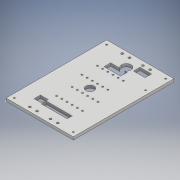
# Autodesk Inventor part: 一枚目2018.8.7
Saved by Autodesk Inventor 2018 (Build 220112000, 112)
## iProperties
Created: 2018-08-07
Part Number: 一枚目2018.8.7
Material: 一般
Document SubType Name: Modeling
Designer: shun2
Density: 1 g/cm^3
Appearance: 既定
Author: shun2
Autodesk Inventor part; units mm, degrees
(part 1 of 2)
ref_plane "YZ Plane" through (0, 0, 0) normal (1, 0, 0) x (0, 1, 0)
ref_plane "XZ Plane" through (0, 0, 0) normal (0, 1, 0) x (-1, 0, 0)
ref_plane "XY Plane" through (0, 0, 0) normal (0, 0, 1) x (1, 0, 0)
sketch "スケッチ1" plane through (0, 0, 0) normal (0, 0, 1) x (1, 0, 0)
  line L0 (0, 0) -> (130, 0)
  line L1 (130, 0) -> (130, 194.7239)
  line L2 (130, 194.7239) -> (0, 194.7239)
  line L3 (0, 194.7239) -> (0, 0)
  circle A0 centre (78, 186.7239) radius 2.15
  circle A1 centre (92, 186.7239) radius 2.15
  circle A2 centre (52, 186.7239) radius 2.15
  circle A3 centre (38, 186.7239) radius 2.15
  circle A4 centre (78, 8) radius 2.15
  circle A5 centre (92, 8) radius 2.15
  circle A6 centre (52, 8) radius 2.15
  circle A7 centre (38, 8) radius 2.15
  circle A8 centre (95.5, 52.362) radius 1.6
  circle A9 centre (45.5, 52.362) radius 1.6
  circle A10 centre (55.5, 52.362) radius 1.6
  circle A11 centre (65.5, 52.362) radius 1.6
  circle A12 centre (75.5, 52.362) radius 1.6
  circle A13 centre (85.5, 52.362) radius 1.6
  circle A14 centre (95.5, 82.362) radius 1.6
  circle A15 centre (45.5, 82.362) radius 1.6
  circle A16 centre (55.5, 82.362) radius 1.6
  circle A17 centre (65.5, 82.362) radius 1.6
  circle A18 centre (75.5, 82.362) radius 1.6
  circle A19 centre (85.5, 82.362) radius 1.6
  circle A20 centre (34.5, 142.362) radius 1.6
  circle A21 centre (84.5, 142.362) radius 1.6
  circle A22 centre (74.5, 142.362) radius 1.6
  circle A23 centre (64.5, 142.362) radius 1.6
  circle A24 centre (54.5, 142.362) radius 1.6
  circle A25 centre (44.5, 142.362) radius 1.6
  circle A26 centre (34.5, 112.362) radius 1.6
  circle A27 centre (84.5, 112.362) radius 1.6
  circle A28 centre (74.5, 112.362) radius 1.6
  circle A29 centre (64.5, 112.362) radius 1.6
  circle A30 centre (54.5, 112.362) radius 1.6
  circle A31 centre (44.5, 112.362) radius 1.6
  circle A32 centre (65, 97.362) radius 8
  arc A33 (69.6765, 160.0343) -> (60.3235, 160.0343) centre (65, 167.7239) ccw
  circle A34 centre (122, 8) radius 1.6
  circle A35 centre (8, 186.7239) radius 1.6
  circle A36 centre (122, 186.7239) radius 1.6
  circle A37 centre (8, 8) radius 1.6
  circle A38 centre (122, 147.7239) radius 1.6
  line L4 (65, 197.7239) -> (65, -3)
  line L5 (-3, 97.362) -> (133, 97.362)
  line L6 (8, 182.1239) -> (8, 191.3239)
  line L7 (117.4, 186.7239) -> (126.6, 186.7239)
  line L8 (122, 182.1239) -> (122, 191.3239)
  line L9 (117.4, 8) -> (126.6, 8)
  line L10 (3.4, 186.7239) -> (12.6, 186.7239)
  line L11 (122, 3.4) -> (122, 12.6)
  line L12 (3.4, 8) -> (12.6, 8)
  line L13 (8, 3.4) -> (8, 12.6)
  line L14 (117.4, 147.7239) -> (126.6, 147.7239)
  line L15 (122, 143.1239) -> (122, 152.3239)
  arc A39 (69.6765, 160.0343) -> (65, 176.7239) centre (65, 167.7239) ccw
  arc A40 (65, 176.7239) -> (60.3235, 160.0343) centre (65, 167.7239) ccw
  line L16 (83.4433, 173.4847) -> (95.4433, 173.4847)
  arc A41 (95.4433, 173.453) -> (95.4433, 173.5164) centre (95.4433, 173.4847) ccw
  arc A42 (83.4433, 173.5164) -> (83.4433, 173.453) centre (83.4433, 173.4847) ccw
  line L17 (95.4433, 173.4847) -> (95.4433, 176.9847)
  arc A43 (95.4751, 176.9847) -> (95.4116, 176.9847) centre (95.4434, 176.9847) ccw
  arc A44 (95.4116, 173.4847) -> (95.4751, 173.4847) centre (95.4434, 173.4847) ccw
  line L18 (95.4433, 176.9847) -> (83.4433, 176.9847)
  arc A45 (83.4433, 177.0164) -> (83.4433, 176.953) centre (83.4433, 176.9847) ccw
  arc A46 (95.4433, 176.953) -> (95.4433, 177.0164) centre (95.4433, 176.9847) ccw
  line L19 (83.4433, 176.9847) -> (83.4433, 173.4847)
  arc A47 (83.4116, 173.4847) -> (83.4751, 173.4847) centre (83.4434, 173.4847) ccw
  arc A48 (83.4751, 176.9847) -> (83.4116, 176.9847) centre (83.4434, 176.9847) ccw
  line L20 (56.515, 150.7744) -> (56.515, 152.1714)
  arc A49 (56.5531, 152.1714) -> (56.4769, 152.1714) centre (56.515, 152.1714) ccw
  arc A50 (56.4769, 150.7744) -> (56.5531, 150.7744) centre (56.515, 150.7744) ccw
  line L21 (46.355, 158.2674) -> (56.515, 158.2674)
  arc A51 (56.515, 158.2293) -> (56.515, 158.3055) centre (56.515, 158.2674) ccw
  arc A52 (46.355, 158.3055) -> (46.355, 158.2293) centre (46.355, 158.2674) ccw
  line L22 (46.355, 158.2674) -> (46.355, 156.4894)
  arc A53 (46.3169, 156.4894) -> (46.3931, 156.4894) centre (46.355, 156.4894) ccw
  arc A54 (46.3931, 158.2674) -> (46.3169, 158.2674) centre (46.355, 158.2674) ccw
  line L23 (56.515, 150.7744) -> (46.355, 150.7744)
  arc A55 (46.355, 150.8125) -> (46.355, 150.7363) centre (46.355, 150.7744) ccw
  arc A56 (56.515, 150.7363) -> (56.515, 150.8125) centre (56.515, 150.7744) ccw
  line L24 (56.515, 157.3784) -> (57.023, 157.5054)
  arc A57 (57.0322, 157.4684) -> (57.0138, 157.5424) centre (57.023, 157.5054) ccw
  arc A58 (56.5058, 157.4154) -> (56.5242, 157.3414) centre (56.515, 157.3784) ccw
  line L25 (56.515, 157.3784) -> (56.515, 158.2674)
  arc A59 (56.5531, 158.2674) -> (56.4769, 158.2674) centre (56.515, 158.2674) ccw
  arc A60 (56.4769, 157.3784) -> (56.5531, 157.3784) centre (56.515, 157.3784) ccw
  line L26 (57.023, 157.5054) -> (57.023, 156.3624)
  arc A61 (56.9849, 156.3624) -> (57.0611, 156.3624) centre (57.023, 156.3624) ccw
  arc A62 (57.0611, 157.5054) -> (56.9849, 157.5054) centre (57.023, 157.5054) ccw
  line L27 (57.023, 156.3624) -> (56.515, 156.4894)
  arc A63 (56.5242, 156.5264) -> (56.5058, 156.4524) centre (56.515, 156.4894) ccw
  arc A64 (57.0138, 156.3254) -> (57.0322, 156.3994) centre (57.023, 156.3624) ccw
  line L28 (56.515, 156.4894) -> (56.515, 157.3784)
  arc A65 (56.5531, 157.3784) -> (56.4769, 157.3784) centre (56.515, 157.3784) ccw
  arc A66 (56.4769, 156.4894) -> (56.5531, 156.4894) centre (56.515, 156.4894) ccw
  line L29 (56.515, 156.4894) -> (46.355, 156.4894)
  arc A67 (46.355, 156.5275) -> (46.355, 156.4513) centre (46.355, 156.4894) ccw
  arc A68 (56.515, 156.4513) -> (56.515, 156.5275) centre (56.515, 156.4894) ccw
  line L30 (46.355, 156.4894) -> (46.355, 152.1714)
  arc A69 (46.3169, 152.1714) -> (46.3931, 152.1714) centre (46.355, 152.1714) ccw
  arc A70 (46.3931, 156.4894) -> (46.3169, 156.4894) centre (46.355, 156.4894) ccw
  line L31 (56.515, 152.1714) -> (46.355, 152.1714)
  arc A71 (46.355, 152.2095) -> (46.355, 152.1333) centre (46.355, 152.1714) ccw
  arc A72 (56.515, 152.1333) -> (56.515, 152.2095) centre (56.515, 152.1714) ccw
  line L32 (56.515, 152.1714) -> (56.515, 156.4894)
  arc A73 (56.5531, 156.4894) -> (56.4769, 156.4894) centre (56.515, 156.4894) ccw
  arc A74 (56.4769, 152.1714) -> (56.5531, 152.1714) centre (56.515, 152.1714) ccw
  line L33 (46.355, 152.1714) -> (46.355, 150.7744)
  arc A75 (46.3169, 150.7744) -> (46.3931, 150.7744) centre (46.355, 150.7744) ccw
  arc A76 (46.3931, 152.1714) -> (46.3169, 152.1714) centre (46.355, 152.1714) ccw
  line L34 (60.565, 151.81) -> (60.565, 156.89)
  arc A77 (60.5968, 156.89) -> (60.5333, 156.89) centre (60.5651, 156.89) ccw
  arc A78 (60.5333, 151.81) -> (60.5968, 151.81) centre (60.5651, 151.81) ccw
  line L35 (60.565, 156.89) -> (61.835, 156.89)
  arc A79 (61.835, 156.8583) -> (61.835, 156.9218) centre (61.835, 156.8901) ccw
  arc A80 (60.565, 156.9218) -> (60.565, 156.8583) centre (60.565, 156.8901) ccw
  line L36 (61.835, 156.89) -> (69.455, 156.89)
  arc A81 (69.455, 156.8583) -> (69.455, 156.9218) centre (69.455, 156.8901) ccw
  arc A82 (61.835, 156.9218) -> (61.835, 156.8583) centre (61.835, 156.8901) ccw
  line L37 (69.455, 156.89) -> (70.725, 156.89)
  arc A83 (70.725, 156.8583) -> (70.725, 156.9218) centre (70.725, 156.8901) ccw
  arc A84 (69.455, 156.9218) -> (69.455, 156.8583) centre (69.455, 156.8901) ccw
  line L38 (70.725, 156.89) -> (70.725, 151.81)
  arc A85 (70.6933, 151.81) -> (70.7568, 151.81) centre (70.725, 151.81) ccw
  arc A86 (70.7568, 156.89) -> (70.6933, 156.89) centre (70.725, 156.89) ccw
  line L39 (70.725, 151.81) -> (60.565, 151.81)
  arc A87 (60.565, 151.8417) -> (60.565, 151.7783) centre (60.565, 151.81) ccw
  arc A88 (70.725, 151.7783) -> (70.725, 151.8417) centre (70.725, 151.81) ccw
  line L40 (61.835, 156.89) -> (61.835, 155.62)
  arc A89 (61.8032, 155.62) -> (61.8668, 155.62) centre (61.835, 155.62) ccw
  arc A90 (61.8668, 156.89) -> (61.8032, 156.89) centre (61.835, 156.89) ccw
  line L41 (61.835, 155.62) -> (69.455, 155.62)
  arc A91 (69.455, 155.5883) -> (69.455, 155.6517) centre (69.455, 155.62) ccw
  arc A92 (61.835, 155.6517) -> (61.835, 155.5883) centre (61.835, 155.62) ccw
  line L42 (69.455, 155.62) -> (69.455, 156.89)
  arc A93 (69.4868, 156.89) -> (69.4232, 156.89) centre (69.455, 156.89) ccw
  arc A94 (69.4232, 155.62) -> (69.4868, 155.62) centre (69.455, 155.62) ccw
  arc A95 (93.9433, 174.5922) -> (93.9433, 175.1172) centre (93.9433, 174.8547) ccw
  arc A96 (93.9433, 175.1172) -> (93.9433, 174.5922) centre (93.9433, 174.8547) ccw
  arc A97 (93.9433, 174.5922) -> (93.9433, 175.1172) centre (93.9433, 174.8547) ccw
  arc A98 (93.9433, 175.1172) -> (93.9433, 174.5922) centre (93.9433, 174.8547) ccw
  arc A99 (92.4433, 174.5922) -> (92.4433, 175.1172) centre (92.4433, 174.8547) ccw
  arc A100 (92.4433, 175.1172) -> (92.4433, 174.5922) centre (92.4433, 174.8547) ccw
  arc A101 (92.4433, 174.5922) -> (92.4433, 175.1172) centre (92.4433, 174.8547) ccw
  arc A102 (92.4433, 175.1172) -> (92.4433, 174.5922) centre (92.4433, 174.8547) ccw
  arc A103 (90.9433, 174.5922) -> (90.9433, 175.1172) centre (90.9433, 174.8547) ccw
  arc A104 (90.9433, 175.1172) -> (90.9433, 174.5922) centre (90.9433, 174.8547) ccw
  arc A105 (90.9433, 174.5922) -> (90.9433, 175.1172) centre (90.9433, 174.8547) ccw
  arc A106 (90.9433, 175.1172) -> (90.9433, 174.5922) centre (90.9433, 174.8547) ccw
  arc A107 (89.4433, 174.5922) -> (89.4433, 175.1172) centre (89.4433, 174.8547) ccw
  arc A108 (89.4433, 175.1172) -> (89.4433, 174.5922) centre (89.4433, 174.8547) ccw
  arc A109 (89.4433, 174.5922) -> (89.4433, 175.1172) centre (89.4433, 174.8547) ccw
  arc A110 (89.4433, 175.1172) -> (89.4433, 174.5922) centre (89.4433, 174.8547) ccw
  arc A111 (87.9433, 174.5922) -> (87.9433, 175.1172) centre (87.9433, 174.8547) ccw
  arc A112 (87.9433, 175.1172) -> (87.9433, 174.5922) centre (87.9433, 174.8547) ccw
  arc A113 (87.9433, 174.5922) -> (87.9433, 175.1172) centre (87.9433, 174.8547) ccw
  arc A114 (87.9433, 175.1172) -> (87.9433, 174.5922) centre (87.9433, 174.8547) ccw
  arc A115 (86.4433, 174.5922) -> (86.4433, 175.1172) centre (86.4433, 174.8547) ccw
  arc A116 (86.4433, 175.1172) -> (86.4433, 174.5922) centre (86.4433, 174.8547) ccw
  arc A117 (86.4433, 174.5922) -> (86.4433, 175.1172) centre (86.4433, 174.8547) ccw
  arc A118 (86.4433, 175.1172) -> (86.4433, 174.5922) centre (86.4433, 174.8547) ccw
  arc A119 (84.9433, 174.5922) -> (84.9433, 175.1172) centre (84.9433, 174.8547) ccw
  arc A120 (84.9433, 175.1172) -> (84.9433, 174.5922) centre (84.9433, 174.8547) ccw
  arc A121 (84.9433, 174.5922) -> (84.9433, 175.1172) centre (84.9433, 174.8547) ccw
  arc A122 (84.9433, 175.1172) -> (84.9433, 174.5922) centre (84.9433, 174.8547) ccw
  line L43 (51.935, 154.8304) -> (50.935, 154.8304)
  line L44 (50.935, 154.8304) -> (50.935, 153.8304)
  line L45 (50.935, 153.8304) -> (51.935, 153.8304)
  line L46 (51.935, 153.8304) -> (51.935, 154.8304)
  line L47 (53.9496, 153.3398) -> (53.9496, 155.321)
  arc A123 (54.4449, 155.321) -> (53.4543, 155.321) centre (53.9496, 155.321) ccw
  arc A124 (53.4543, 153.3398) -> (54.4449, 153.3398) centre (53.9496, 153.3398) ccw
  line L48 (53.9496, 153.3398) -> (53.9496, 155.321)
  arc A125 (54.4449, 155.321) -> (53.4543, 155.321) centre (53.9496, 155.321) ccw
  arc A126 (53.4543, 153.3398) -> (54.4449, 153.3398) centre (53.9496, 153.3398) ccw
  line L49 (48.9204, 153.3398) -> (48.9204, 155.321)
  arc A127 (49.4157, 155.321) -> (48.4251, 155.321) centre (48.9204, 155.321) ccw
  arc A128 (48.4251, 153.3398) -> (49.4157, 153.3398) centre (48.9204, 153.3398) ccw
  line L50 (48.9204, 153.3398) -> (48.9204, 155.321)
  arc A129 (49.4157, 155.321) -> (48.4251, 155.321) centre (48.9204, 155.321) ccw
  arc A130 (48.4251, 153.3398) -> (49.4157, 153.3398) centre (48.9204, 153.3398) ccw
  arc A131 (63.105, 153.9) -> (63.105, 154.8) centre (63.105, 154.35) ccw
  arc A132 (63.105, 154.8) -> (63.105, 153.9) centre (63.105, 154.35) ccw
  arc A133 (63.105, 153.9) -> (63.105, 154.8) centre (63.105, 154.35) ccw
  arc A134 (63.105, 154.8) -> (63.105, 153.9) centre (63.105, 154.35) ccw
  arc A135 (65.645, 153.9) -> (65.645, 154.8) centre (65.645, 154.35) ccw
  arc A136 (65.645, 154.8) -> (65.645, 153.9) centre (65.645, 154.35) ccw
  arc A137 (65.645, 153.9) -> (65.645, 154.8) centre (65.645, 154.35) ccw
  arc A138 (65.645, 154.8) -> (65.645, 153.9) centre (65.645, 154.35) ccw
  arc A139 (68.185, 153.9) -> (68.185, 154.8) centre (68.185, 154.35) ccw
  arc A140 (68.185, 154.8) -> (68.185, 153.9) centre (68.185, 154.35) ccw
  arc A141 (68.185, 153.9) -> (68.185, 154.8) centre (68.185, 154.35) ccw
  arc A142 (68.185, 154.8) -> (68.185, 153.9) centre (68.185, 154.35) ccw
  line L51 (74.3631, 160.0343) -> (74.3631, 147.2613)
  line L52 (74.3631, 147.2613) -> (42.3354, 147.2613)
  line L53 (42.3354, 147.2613) -> (42.3354, 160.0343)
  line L54 (78, 180.9909) -> (100.5174, 180.9909)
  line L55 (100.5174, 180.9909) -> (100.5174, 168.379)
  line L56 (100.5174, 168.379) -> (78, 168.379)
  line L57 (78, 168.379) -> (78, 180.9909)
  arc A143 (69.6765, 160.0343) -> (60.3235, 160.0343) centre (65, 167.7239) ccw
  line L58 (42.3354, 160.0343) -> (60.3235, 160.0343)
  line L59 (69.6765, 160.0343) -> (74.3631, 160.0343)
  line L60 (89.7664, 26.5952) -> (89.6098, 26.5952)
  arc A144 (89.6098, 26.6143) -> (89.6098, 26.5762) centre (89.6098, 26.5953) ccw
  arc A145 (89.7664, 26.5762) -> (89.7664, 26.6143) centre (89.7664, 26.5953) ccw
  line L61 (89.6098, 26.5952) -> (89.6098, 26.0731)
  arc A146 (89.5907, 26.0731) -> (89.6288, 26.0731) centre (89.6097, 26.0731) ccw
  arc A147 (89.6288, 26.5952) -> (89.5907, 26.5952) centre (89.6097, 26.5952) ccw
  line L62 (89.6098, 26.0731) -> (89.9231, 26.0731)
  arc A148 (89.9231, 26.0541) -> (89.9231, 26.0922) centre (89.9231, 26.0731) ccw
  arc A149 (89.6098, 26.0922) -> (89.6098, 26.0541) centre (89.6098, 26.0731) ccw
  arc A150 (89.9231, 26.0731) -> (90.1319, 26.2819) centre (89.9231, 26.2819) ccw
  arc A151 (89.9231, 26.0922) -> (89.9231, 26.0541) centre (89.9231, 26.0731) ccw
  arc A152 (90.1509, 26.2819) -> (90.1129, 26.2819) centre (90.1319, 26.2819) ccw
  line L63 (90.1319, 26.2819) -> (90.1319, 26.8041)
  arc A153 (90.1509, 26.8041) -> (90.1129, 26.8041) centre (90.1319, 26.8041) ccw
  arc A154 (90.1129, 26.2819) -> (90.1509, 26.2819) centre (90.1319, 26.2819) ccw
  arc A155 (90.1319, 26.8041) -> (89.9231, 27.0129) centre (89.9231, 26.8041) ccw
  arc A156 (90.1129, 26.8041) -> (90.1509, 26.8041) centre (90.1319, 26.8041) ccw
  arc A157 (89.9231, 27.0319) -> (89.9231, 26.9938) centre (89.9231, 27.0129) ccw
  line L64 (89.9231, 27.0129) -> (89.6098, 27.0129)
  arc A158 (89.6098, 27.032) -> (89.6098, 26.9939) centre (89.6098, 27.013) ccw
  arc A159 (89.9231, 26.9939) -> (89.9231, 27.032) centre (89.9231, 27.013) ccw
  arc A160 (84.5298, 26.2819) -> (84.7386, 26.0731) centre (84.7386, 26.2819) ccw
  arc A161 (84.5488, 26.2819) -> (84.5107, 26.2819) centre (84.5298, 26.2819) ccw
  arc A162 (84.7386, 26.0541) -> (84.7386, 26.0922) centre (84.7386, 26.0731) ccw
  arc A163 (84.7386, 26.0731) -> (85.0519, 26.2036) centre (84.7387, 26.5143) ccw
  arc A164 (84.7386, 26.0921) -> (84.7386, 26.0541) centre (84.7386, 26.0731) ccw
  arc A165 (85.0654, 26.1902) -> (85.0384, 26.217) centre (85.0519, 26.2036) ccw
  arc A166 (85.0258, 26.8041) -> (84.817, 27.0129) centre (84.817, 26.8041) ccw
  arc A167 (85.0067, 26.8041) -> (85.0448, 26.8041) centre (85.0257, 26.8041) ccw
  arc A168 (84.817, 27.032) -> (84.817, 26.9939) centre (84.817, 27.013) ccw
  arc A169 (84.817, 27.0129) -> (84.582, 26.9346) centre (84.8169, 26.6213) ccw
  arc A170 (84.817, 26.9939) -> (84.8169, 27.032) centre (84.817, 27.013) ccw
  arc A171 (84.5706, 26.9498) -> (84.5934, 26.9193) centre (84.582, 26.9346) ccw
  arc A172 (84.9214, 26.6213) -> (85.0258, 26.8041) centre (84.8137, 26.804) ccw
  arc A173 (84.9117, 26.6377) -> (84.931, 26.6049) centre (84.9213, 26.6213) ccw
  arc A174 (85.0448, 26.8041) -> (85.0067, 26.8041) centre (85.0257, 26.8041) ccw
  arc A175 (84.6342, 26.4647) -> (84.5298, 26.2819) centre (84.7419, 26.282) ccw
  arc A176 (84.6439, 26.4483) -> (84.6245, 26.4811) centre (84.6342, 26.4647) ccw
  arc A177 (84.5107, 26.2819) -> (84.5488, 26.2819) centre (84.5298, 26.2819) ccw
  line L65 (84.6342, 26.4647) -> (84.9214, 26.6213)
  arc A178 (84.9305, 26.6046) -> (84.9123, 26.638) centre (84.9214, 26.6213) ccw
  arc A179 (84.6251, 26.4814) -> (84.6433, 26.448) centre (84.6342, 26.4647) ccw
  line L66 (84.0898, 27.0129) -> (84.0898, 26.0731)
  arc A180 (84.0708, 26.0731) -> (84.1089, 26.0731) centre (84.0899, 26.0731) ccw
  arc A181 (84.1089, 27.0129) -> (84.0708, 27.0129) centre (84.0899, 27.0129) ccw
  line L67 (84.1942, 26.0731) -> (83.9854, 26.0731)
  arc A182 (83.9854, 26.0922) -> (83.9854, 26.0541) centre (83.9854, 26.0731) ccw
  arc A183 (84.1942, 26.0541) -> (84.1942, 26.0922) centre (84.1942, 26.0731) ccw
  line L68 (84.1942, 27.0129) -> (83.9854, 27.0129)
  arc A184 (83.9854, 27.032) -> (83.9854, 26.9939) centre (83.9854, 27.013) ccw
  arc A185 (84.1942, 26.9939) -> (84.1942, 27.032) centre (84.1942, 27.013) ccw
  line L69 (83.2234, 26.5952) -> (83.0668, 26.5952)
  arc A186 (83.0668, 26.6143) -> (83.0668, 26.5762) centre (83.0668, 26.5953) ccw
  arc A187 (83.2234, 26.5762) -> (83.2234, 26.6143) centre (83.2234, 26.5953) ccw
  line L70 (83.0668, 26.5952) -> (83.0668, 26.0731)
  arc A188 (83.0477, 26.0731) -> (83.0858, 26.0731) centre (83.0668, 26.0731) ccw
  arc A189 (83.0858, 26.5952) -> (83.0477, 26.5952) centre (83.0668, 26.5952) ccw
  line L71 (83.0668, 26.0731) -> (83.38, 26.0731)
  arc A190 (83.38, 26.0541) -> (83.38, 26.0922) centre (83.38, 26.0731) ccw
  arc A191 (83.0668, 26.0922) -> (83.0668, 26.0541) centre (83.0668, 26.0731) ccw
  arc A192 (83.38, 26.0731) -> (83.5889, 26.2819) centre (83.38, 26.282) ccw
  arc A193 (83.38, 26.0922) -> (83.38, 26.0541) centre (83.38, 26.0731) ccw
  arc A194 (83.6079, 26.2819) -> (83.5698, 26.2819) centre (83.5889, 26.2819) ccw
  line L72 (83.5889, 26.2819) -> (83.5889, 26.8041)
  arc A195 (83.6079, 26.8041) -> (83.5698, 26.8041) centre (83.5889, 26.8041) ccw
  arc A196 (83.5698, 26.2819) -> (83.6079, 26.2819) centre (83.5889, 26.2819) ccw
  arc A197 (83.5889, 26.8041) -> (83.38, 27.0129) centre (83.38, 26.804) ccw
  arc A198 (83.5698, 26.8041) -> (83.6079, 26.8041) centre (83.5889, 26.8041) ccw
  arc A199 (83.38, 27.0319) -> (83.38, 26.9938) centre (83.38, 27.0129) ccw
  line L73 (83.38, 27.0129) -> (83.0668, 27.0129)
  arc A200 (83.0668, 27.032) -> (83.0668, 26.9939) centre (83.0668, 27.013) ccw
  arc A201 (83.38, 26.9939) -> (83.38, 27.032) centre (83.38, 27.013) ccw
  line L74 (31.115, 35.941) -> (31.115, 34.544)
  arc A202 (31.0769, 34.544) -> (31.1531, 34.544) centre (31.115, 34.544) ccw
  arc A203 (31.1531, 35.941) -> (31.0769, 35.941) centre (31.115, 35.941) ccw
  line L75 (41.275, 28.448) -> (31.115, 28.448)
  arc A204 (31.115, 28.4861) -> (31.115, 28.4099) centre (31.115, 28.448) ccw
  arc A205 (41.275, 28.4099) -> (41.275, 28.4861) centre (41.275, 28.448) ccw
  line L76 (41.275, 28.448) -> (41.275, 30.226)
  arc A206 (41.3131, 30.226) -> (41.2369, 30.226) centre (41.275, 30.226) ccw
  arc A207 (41.2369, 28.448) -> (41.3131, 28.448) centre (41.275, 28.448) ccw
  line L77 (31.115, 35.941) -> (41.275, 35.941)
  arc A208 (41.275, 35.9029) -> (41.275, 35.9791) centre (41.275, 35.941) ccw
  arc A209 (31.115, 35.9791) -> (31.115, 35.9029) centre (31.115, 35.941) ccw
  line L78 (31.115, 29.337) -> (30.607, 29.21)
  arc A210 (30.5978, 29.247) -> (30.6162, 29.173) centre (30.607, 29.21) ccw
  arc A211 (31.1242, 29.3) -> (31.1058, 29.374) centre (31.115, 29.337) ccw
  line L79 (31.115, 29.337) -> (31.115, 28.448)
  arc A212 (31.0769, 28.448) -> (31.1531, 28.448) centre (31.115, 28.448) ccw
  arc A213 (31.1531, 29.337) -> (31.0769, 29.337) centre (31.115, 29.337) ccw
  line L80 (30.607, 29.21) -> (30.607, 30.353)
  arc A214 (30.6451, 30.353) -> (30.5689, 30.353) centre (30.607, 30.353) ccw
  arc A215 (30.5689, 29.21) -> (30.6451, 29.21) centre (30.607, 29.21) ccw
  line L81 (30.607, 30.353) -> (31.115, 30.226)
  arc A216 (31.1058, 30.189) -> (31.1242, 30.263) centre (31.115, 30.226) ccw
  arc A217 (30.6162, 30.39) -> (30.5978, 30.316) centre (30.607, 30.353) ccw
  line L82 (31.115, 30.226) -> (31.115, 29.337)
  arc A218 (31.0769, 29.337) -> (31.1531, 29.337) centre (31.115, 29.337) ccw
  arc A219 (31.1531, 30.226) -> (31.0769, 30.226) centre (31.115, 30.226) ccw
  line L83 (31.115, 30.226) -> (41.275, 30.226)
  arc A220 (41.275, 30.1879) -> (41.275, 30.2641) centre (41.275, 30.226) ccw
  arc A221 (31.115, 30.2641) -> (31.115, 30.1879) centre (31.115, 30.226) ccw
  line L84 (41.275, 30.226) -> (41.275, 34.544)
  arc A222 (41.3131, 34.544) -> (41.2369, 34.544) centre (41.275, 34.544) ccw
  arc A223 (41.2369, 30.226) -> (41.3131, 30.226) centre (41.275, 30.226) ccw
  line L85 (31.115, 34.544) -> (41.275, 34.544)
  arc A224 (41.275, 34.5059) -> (41.275, 34.5821) centre (41.275, 34.544) ccw
  arc A225 (31.115, 34.5821) -> (31.115, 34.5059) centre (31.115, 34.544) ccw
  line L86 (31.115, 34.544) -> (31.115, 30.226)
  arc A226 (31.0769, 30.226) -> (31.1531, 30.226) centre (31.115, 30.226) ccw
  arc A227 (31.1531, 34.544) -> (31.0769, 34.544) centre (31.115, 34.544) ccw
  line L87 (41.275, 34.544) -> (41.275, 35.941)
  arc A228 (41.3131, 35.941) -> (41.2369, 35.941) centre (41.275, 35.941) ccw
  arc A229 (41.2369, 34.544) -> (41.3131, 34.544) centre (41.275, 34.544) ccw
  line L88 (32.2933, 29.5896) -> (32.0534, 29.7815)
  arc A230 (32.0732, 29.8063) -> (32.0336, 29.7567) centre (32.0534, 29.7815) ccw
  arc A231 (32.2734, 29.5648) -> (32.3131, 29.6144) centre (32.2933, 29.5896) ccw
  line L89 (32.0534, 29.7815) -> (32.0534, 28.9179)
  arc A232 (32.0216, 28.9179) -> (32.0851, 28.9179) centre (32.0533, 28.9179) ccw
  arc A233 (32.0851, 29.7815) -> (32.0216, 29.7815) centre (32.0533, 29.7815) ccw
  line L90 (32.2933, 28.9179) -> (31.8135, 28.9179)
  arc A234 (31.8135, 28.9497) -> (31.8135, 28.8862) centre (31.8135, 28.918) ccw
  arc A235 (32.2933, 28.8862) -> (32.2933, 28.9497) centre (32.2933, 28.918) ccw
  arc A236 (37.1094, 29.7815) -> (36.8935, 29.5656) centre (37.1094, 29.5656) ccw
  arc A237 (37.1094, 29.7498) -> (37.1094, 29.8133) centre (37.1094, 29.7816) ccw
  arc A238 (36.8618, 29.5656) -> (36.9253, 29.5656) centre (36.8936, 29.5656) ccw
  arc A239 (37.3733, 29.5896) -> (37.1094, 29.7815) centre (37.1094, 29.5041) ccw
  arc A240 (37.3431, 29.5798) -> (37.4035, 29.5994) centre (37.3733, 29.5896) ccw
  arc A241 (37.1094, 29.8132) -> (37.1094, 29.7498) centre (37.1094, 29.7815) ccw
  arc A242 (36.8935, 29.5656) -> (36.9655, 29.3977) centre (37.1253, 29.5656) ccw
  arc A243 (36.9252, 29.5656) -> (36.8618, 29.5656) centre (36.8935, 29.5656) ccw
  arc A244 (36.9436, 29.3747) -> (36.9874, 29.4207) centre (36.9655, 29.3977) ccw
  line L91 (36.9655, 29.3977) -> (37.3733, 28.9179)
  arc A245 (37.3491, 28.8973) -> (37.3975, 28.9385) centre (37.3733, 28.9179) ccw
  arc A246 (36.9897, 29.4182) -> (36.9413, 29.3771) centre (36.9655, 29.3976) ccw
  line L92 (37.3733, 28.9179) -> (36.8935, 28.9179)
  arc A247 (36.8935, 28.9497) -> (36.8935, 28.8862) centre (36.8935, 28.918) ccw
  arc A248 (37.3733, 28.8862) -> (37.3733, 28.9497) centre (37.3733, 28.918) ccw
  arc A249 (38.7096, 28.829) -> (38.7096, 29.845) centre (38.7096, 29.337) ccw
  arc A250 (38.7096, 29.845) -> (38.7096, 28.829) centre (38.7096, 29.337) ccw
  arc A251 (33.6804, 28.829) -> (33.6804, 29.845) centre (33.6804, 29.337) ccw
  arc A252 (33.6804, 29.845) -> (33.6804, 28.829) centre (33.6804, 29.337) ccw
  line L93 (47.085, 27.46) -> (48.355, 27.46)
  arc A253 (48.355, 27.4219) -> (48.355, 27.4981) centre (48.355, 27.46) ccw
  arc A254 (47.085, 27.4981) -> (47.085, 27.4219) centre (47.085, 27.46) ccw
  line L94 (48.355, 27.46) -> (48.99, 28.095)
  arc A255 (49.0169, 28.0681) -> (48.9631, 28.1219) centre (48.99, 28.095) ccw
  arc A256 (48.3281, 27.4869) -> (48.3819, 27.4331) centre (48.355, 27.46) ccw
  line L95 (48.99, 29.365) -> (48.355, 30)
  arc A257 (48.3819, 30.0269) -> (48.3281, 29.9731) centre (48.355, 30) ccw
  arc A258 (48.9631, 29.3381) -> (49.0169, 29.3919) centre (48.99, 29.365) ccw
  line L96 (48.99, 28.095) -> (49.625, 27.46)
  arc A259 (49.5981, 27.4331) -> (49.6519, 27.4869) centre (49.625, 27.46) ccw
  arc A260 (49.0169, 28.1219) -> (48.9631, 28.0681) centre (48.99, 28.095) ccw
  line L97 (49.625, 27.46) -> (50.895, 27.46)
  arc A261 (50.895, 27.4219) -> (50.895, 27.4981) centre (50.895, 27.46) ccw
  arc A262 (49.625, 27.4981) -> (49.625, 27.4219) centre (49.625, 27.46) ccw
  line L98 (50.895, 27.46) -> (51.53, 28.095)
  arc A263 (51.5569, 28.0681) -> (51.5031, 28.1219) centre (51.53, 28.095) ccw
  arc A264 (50.8681, 27.4869) -> (50.9219, 27.4331) centre (50.895, 27.46) ccw
  line L99 (51.53, 29.365) -> (50.895, 30)
  arc A265 (50.9219, 30.0269) -> (50.8681, 29.9731) centre (50.895, 30) ccw
  arc A266 (51.5031, 29.3381) -> (51.5569, 29.3919) centre (51.53, 29.365) ccw
  line L100 (50.895, 30) -> (49.625, 30)
  arc A267 (49.625, 30.0381) -> (49.625, 29.9619) centre (49.625, 30) ccw
  arc A268 (50.895, 29.9619) -> (50.895, 30.0381) centre (50.895, 30) ccw
  line L101 (49.625, 30) -> (48.99, 29.365)
  arc A269 (48.9631, 29.3919) -> (49.0169, 29.3381) centre (48.99, 29.365) ccw
  arc A270 (49.6519, 29.9731) -> (49.5981, 30.0269) centre (49.625, 30) ccw
  line L102 (46.45, 28.095) -> (46.45, 29.365)
  arc A271 (46.4881, 29.365) -> (46.4119, 29.365) centre (46.45, 29.365) ccw
  arc A272 (46.4119, 28.095) -> (46.4881, 28.095) centre (46.45, 28.095) ccw
  line L103 (47.085, 27.46) -> (46.45, 28.095)
  arc A273 (46.4769, 28.1219) -> (46.4231, 28.0681) centre (46.45, 28.095) ccw
  arc A274 (47.0581, 27.4331) -> (47.1119, 27.4869) centre (47.085, 27.46) ccw
  line L104 (46.45, 29.365) -> (47.085, 30)
  arc A275 (47.1119, 29.9731) -> (47.0581, 30.0269) centre (47.085, 30) ccw
  arc A276 (46.4231, 29.3919) -> (46.4769, 29.3381) centre (46.45, 29.365) ccw
  line L105 (48.355, 30) -> (47.085, 30)
  arc A277 (47.085, 30.0381) -> (47.085, 29.9619) centre (47.085, 30) ccw
  arc A278 (48.355, 29.9619) -> (48.355, 30.0381) centre (48.355, 30) ccw
  line L106 (51.53, 28.095) -> (52.165, 27.46)
  arc A279 (52.1381, 27.4331) -> (52.1919, 27.4869) centre (52.165, 27.46) ccw
  arc A280 (51.5569, 28.1219) -> (51.5031, 28.0681) centre (51.53, 28.095) ccw
  line L107 (52.165, 27.46) -> (53.435, 27.46)
  arc A281 (53.435, 27.4219) -> (53.435, 27.4981) centre (53.435, 27.46) ccw
  arc A282 (52.165, 27.4981) -> (52.165, 27.4219) centre (52.165, 27.46) ccw
  line L108 (53.435, 27.46) -> (54.07, 28.095)
  arc A283 (54.0969, 28.0681) -> (54.0431, 28.1219) centre (54.07, 28.095) ccw
  arc A284 (53.4081, 27.4869) -> (53.4619, 27.4331) centre (53.435, 27.46) ccw
  line L109 (54.07, 29.365) -> (53.435, 30)
  arc A285 (53.4619, 30.0269) -> (53.4081, 29.9731) centre (53.435, 30) ccw
  arc A286 (54.0431, 29.3381) -> (54.0969, 29.3919) centre (54.07, 29.365) ccw
  line L110 (53.435, 30) -> (52.165, 30)
  arc A287 (52.165, 30.0381) -> (52.165, 29.9619) centre (52.165, 30) ccw
  arc A288 (53.435, 29.9619) -> (53.435, 30.0381) centre (53.435, 30) ccw
  line L111 (52.165, 30) -> (51.53, 29.365)
  arc A289 (51.5031, 29.3919) -> (51.5569, 29.3381) centre (51.53, 29.365) ccw
  arc A290 (52.1919, 29.9731) -> (52.1381, 30.0269) centre (52.165, 30) ccw
  line L112 (54.705, 27.46) -> (55.975, 27.46)
  arc A291 (55.975, 27.4219) -> (55.975, 27.4981) centre (55.975, 27.46) ccw
  arc A292 (54.705, 27.4981) -> (54.705, 27.4219) centre (54.705, 27.46) ccw
  line L113 (55.975, 27.46) -> (56.61, 28.095)
  arc A293 (56.6369, 28.0681) -> (56.5831, 28.1219) centre (56.61, 28.095) ccw
  arc A294 (55.9481, 27.4869) -> (56.0019, 27.4331) centre (55.975, 27.46) ccw
  line L114 (56.61, 29.365) -> (55.975, 30)
  arc A295 (56.0019, 30.0269) -> (55.9481, 29.9731) centre (55.975, 30) ccw
  arc A296 (56.5831, 29.3381) -> (56.6369, 29.3919) centre (56.61, 29.365) ccw
  line L115 (56.61, 28.095) -> (57.245, 27.46)
  arc A297 (57.2181, 27.4331) -> (57.2719, 27.4869) centre (57.245, 27.46) ccw
  arc A298 (56.6369, 28.1219) -> (56.5831, 28.0681) centre (56.61, 28.095) ccw
  line L116 (57.245, 27.46) -> (58.515, 27.46)
  arc A299 (58.515, 27.4219) -> (58.515, 27.4981) centre (58.515, 27.46) ccw
  arc A300 (57.245, 27.4981) -> (57.245, 27.4219) centre (57.245, 27.46) ccw
  line L117 (58.515, 27.46) -> (59.15, 28.095)
  arc A301 (59.1769, 28.0681) -> (59.1231, 28.1219) centre (59.15, 28.095) ccw
  arc A302 (58.4881, 27.4869) -> (58.5419, 27.4331) centre (58.515, 27.46) ccw
  line L118 (59.15, 29.365) -> (58.515, 30)
  arc A303 (58.5419, 30.0269) -> (58.4881, 29.9731) centre (58.515, 30) ccw
  arc A304 (59.1231, 29.3381) -> (59.1769, 29.3919) centre (59.15, 29.365) ccw
  line L119 (58.515, 30) -> (57.245, 30)
  arc A305 (57.245, 30.0381) -> (57.245, 29.9619) centre (57.245, 30) ccw
  arc A306 (58.515, 29.9619) -> (58.515, 30.0381) centre (58.515, 30) ccw
  line L120 (57.245, 30) -> (56.61, 29.365)
  arc A307 (56.5831, 29.3919) -> (56.6369, 29.3381) centre (56.61, 29.365) ccw
  arc A308 (57.2719, 29.9731) -> (57.2181, 30.0269) centre (57.245, 30) ccw
  line L121 (54.705, 27.46) -> (54.07, 28.095)
  arc A309 (54.0969, 28.1219) -> (54.0431, 28.0681) centre (54.07, 28.095) ccw
  arc A310 (54.6781, 27.4331) -> (54.7319, 27.4869) centre (54.705, 27.46) ccw
  line L122 (54.07, 29.365) -> (54.705, 30)
  arc A311 (54.7319, 29.9731) -> (54.6781, 30.0269) centre (54.705, 30) ccw
  arc A312 (54.0431, 29.3919) -> (54.0969, 29.3381) centre (54.07, 29.365) ccw
  line L123 (55.975, 30) -> (54.705, 30)
  arc A313 (54.705, 30.0381) -> (54.705, 29.9619) centre (54.705, 30) ccw
  arc A314 (55.975, 29.9619) -> (55.975, 30.0381) centre (55.975, 30) ccw
  line L124 (59.15, 28.095) -> (59.785, 27.46)
  arc A315 (59.7581, 27.4331) -> (59.8119, 27.4869) centre (59.785, 27.46) ccw
  arc A316 (59.1769, 28.1219) -> (59.1231, 28.0681) centre (59.15, 28.095) ccw
  line L125 (59.785, 27.46) -> (61.055, 27.46)
  arc A317 (61.055, 27.4219) -> (61.055, 27.4981) centre (61.055, 27.46) ccw
  arc A318 (59.785, 27.4981) -> (59.785, 27.4219) centre (59.785, 27.46) ccw
  line L126 (61.055, 27.46) -> (61.69, 28.095)
  arc A319 (61.7169, 28.0681) -> (61.6631, 28.1219) centre (61.69, 28.095) ccw
  arc A320 (61.0281, 27.4869) -> (61.0819, 27.4331) centre (61.055, 27.46) ccw
  line L127 (61.69, 29.365) -> (61.055, 30)
  arc A321 (61.0819, 30.0269) -> (61.0281, 29.9731) centre (61.055, 30) ccw
  arc A322 (61.6631, 29.3381) -> (61.7169, 29.3919) centre (61.69, 29.365) ccw
  line L128 (61.055, 30) -> (59.785, 30)
  arc A323 (59.785, 30.0381) -> (59.785, 29.9619) centre (59.785, 30) ccw
  arc A324 (61.055, 29.9619) -> (61.055, 30.0381) centre (61.055, 30) ccw
  line L129 (59.785, 30) -> (59.15, 29.365)
  arc A325 (59.1231, 29.3919) -> (59.1769, 29.3381) centre (59.15, 29.365) ccw
  arc A326 (59.8119, 29.9731) -> (59.7581, 30.0269) centre (59.785, 30) ccw
  line L130 (62.325, 27.46) -> (63.595, 27.46)
  arc A327 (63.595, 27.4219) -> (63.595, 27.4981) centre (63.595, 27.46) ccw
  arc A328 (62.325, 27.4981) -> (62.325, 27.4219) centre (62.325, 27.46) ccw
  line L131 (63.595, 27.46) -> (64.23, 28.095)
  arc A329 (64.2569, 28.0681) -> (64.2031, 28.1219) centre (64.23, 28.095) ccw
  arc A330 (63.5681, 27.4869) -> (63.6219, 27.4331) centre (63.595, 27.46) ccw
  line L132 (64.23, 29.365) -> (63.595, 30)
  arc A331 (63.6219, 30.0269) -> (63.5681, 29.9731) centre (63.595, 30) ccw
  arc A332 (64.2031, 29.3381) -> (64.2569, 29.3919) centre (64.23, 29.365) ccw
  line L133 (64.23, 28.095) -> (64.865, 27.46)
  arc A333 (64.8381, 27.4331) -> (64.8919, 27.4869) centre (64.865, 27.46) ccw
  arc A334 (64.2569, 28.1219) -> (64.2031, 28.0681) centre (64.23, 28.095) ccw
  line L134 (64.865, 27.46) -> (66.135, 27.46)
  arc A335 (66.135, 27.4219) -> (66.135, 27.4981) centre (66.135, 27.46) ccw
  arc A336 (64.865, 27.4981) -> (64.865, 27.4219) centre (64.865, 27.46) ccw
  line L135 (66.135, 27.46) -> (66.77, 28.095)
  arc A337 (66.7969, 28.0681) -> (66.7431, 28.1219) centre (66.77, 28.095) ccw
  arc A338 (66.1081, 27.4869) -> (66.1619, 27.4331) centre (66.135, 27.46) ccw
  line L136 (66.77, 29.365) -> (66.135, 30)
  arc A339 (66.1619, 30.0269) -> (66.1081, 29.9731) centre (66.135, 30) ccw
  arc A340 (66.7431, 29.3381) -> (66.7969, 29.3919) centre (66.77, 29.365) ccw
  line L137 (66.135, 30) -> (64.865, 30)
  arc A341 (64.865, 30.0381) -> (64.865, 29.9619) centre (64.865, 30) ccw
  arc A342 (66.135, 29.9619) -> (66.135, 30.0381) centre (66.135, 30) ccw
  line L138 (64.865, 30) -> (64.23, 29.365)
  arc A343 (64.2031, 29.3919) -> (64.2569, 29.3381) centre (64.23, 29.365) ccw
  arc A344 (64.8919, 29.9731) -> (64.8381, 30.0269) centre (64.865, 30) ccw
  line L139 (62.325, 27.46) -> (61.69, 28.095)
  arc A345 (61.7169, 28.1219) -> (61.6631, 28.0681) centre (61.69, 28.095) ccw
  arc A346 (62.2981, 27.4331) -> (62.3519, 27.4869) centre (62.325, 27.46) ccw
  line L140 (61.69, 29.365) -> (62.325, 30)
  arc A347 (62.3519, 29.9731) -> (62.2981, 30.0269) centre (62.325, 30) ccw
  arc A348 (61.6631, 29.3919) -> (61.7169, 29.3381) centre (61.69, 29.365) ccw
  line L141 (63.595, 30) -> (62.325, 30)
  arc A349 (62.325, 30.0381) -> (62.325, 29.9619) centre (62.325, 30) ccw
  arc A350 (63.595, 29.9619) -> (63.595, 30.0381) centre (63.595, 30) ccw
  line L142 (66.77, 28.095) -> (67.405, 27.46)
  arc A351 (67.3781, 27.4331) -> (67.4319, 27.4869) centre (67.405, 27.46) ccw
  arc A352 (66.7969, 28.1219) -> (66.7431, 28.0681) centre (66.77, 28.095) ccw
  line L143 (67.405, 27.46) -> (68.675, 27.46)
  arc A353 (68.675, 27.4219) -> (68.675, 27.4981) centre (68.675, 27.46) ccw
  arc A354 (67.405, 27.4981) -> (67.405, 27.4219) centre (67.405, 27.46) ccw
  line L144 (68.675, 27.46) -> (69.31, 28.095)
  arc A355 (69.3369, 28.0681) -> (69.2831, 28.1219) centre (69.31, 28.095) ccw
  arc A356 (68.6481, 27.4869) -> (68.7019, 27.4331) centre (68.675, 27.46) ccw
  line L145 (69.31, 29.365) -> (68.675, 30)
  arc A357 (68.7019, 30.0269) -> (68.6481, 29.9731) centre (68.675, 30) ccw
  arc A358 (69.2831, 29.3381) -> (69.3369, 29.3919) centre (69.31, 29.365) ccw
  line L146 (68.675, 30) -> (67.405, 30)
  arc A359 (67.405, 30.0381) -> (67.405, 29.9619) centre (67.405, 30) ccw
  arc A360 (68.675, 29.9619) -> (68.675, 30.0381) centre (68.675, 30) ccw
  line L147 (67.405, 30) -> (66.77, 29.365)
  arc A361 (66.7431, 29.3919) -> (66.7969, 29.3381) centre (66.77, 29.365) ccw
  arc A362 (67.4319, 29.9731) -> (67.3781, 30.0269) centre (67.405, 30) ccw
  line L148 (69.945, 27.46) -> (71.215, 27.46)
  arc A363 (71.215, 27.4219) -> (71.215, 27.4981) centre (71.215, 27.46) ccw
  arc A364 (69.945, 27.4981) -> (69.945, 27.4219) centre (69.945, 27.46) ccw
  line L149 (71.215, 27.46) -> (71.85, 28.095)
  arc A365 (71.8769, 28.0681) -> (71.8231, 28.1219) centre (71.85, 28.095) ccw
  arc A366 (71.1881, 27.4869) -> (71.2419, 27.4331) centre (71.215, 27.46) ccw
  line L150 (71.85, 29.365) -> (71.215, 30)
  arc A367 (71.2419, 30.0269) -> (71.1881, 29.9731) centre (71.215, 30) ccw
  arc A368 (71.8231, 29.3381) -> (71.8769, 29.3919) centre (71.85, 29.365) ccw
  line L151 (71.85, 28.095) -> (72.485, 27.46)
  arc A369 (72.4581, 27.4331) -> (72.5119, 27.4869) centre (72.485, 27.46) ccw
  arc A370 (71.8769, 28.1219) -> (71.8231, 28.0681) centre (71.85, 28.095) ccw
  line L152 (72.485, 27.46) -> (73.755, 27.46)
  arc A371 (73.755, 27.4219) -> (73.755, 27.4981) centre (73.755, 27.46) ccw
  arc A372 (72.485, 27.4981) -> (72.485, 27.4219) centre (72.485, 27.46) ccw
  line L153 (73.755, 27.46) -> (74.39, 28.095)
  arc A373 (74.4169, 28.0681) -> (74.3631, 28.1219) centre (74.39, 28.095) ccw
  arc A374 (73.7281, 27.4869) -> (73.7819, 27.4331) centre (73.755, 27.46) ccw
  line L154 (74.39, 29.365) -> (73.755, 30)
  arc A375 (73.7819, 30.0269) -> (73.7281, 29.9731) centre (73.755, 30) ccw
  arc A376 (74.3631, 29.3381) -> (74.4169, 29.3919) centre (74.39, 29.365) ccw
  line L155 (73.755, 30) -> (72.485, 30)
  arc A377 (72.485, 30.0381) -> (72.485, 29.9619) centre (72.485, 30) ccw
  arc A378 (73.755, 29.9619) -> (73.755, 30.0381) centre (73.755, 30) ccw
  line L156 (72.485, 30) -> (71.85, 29.365)
  arc A379 (71.8231, 29.3919) -> (71.8769, 29.3381) centre (71.85, 29.365) ccw
  arc A380 (72.5119, 29.9731) -> (72.4581, 30.0269) centre (72.485, 30) ccw
  line L157 (69.945, 27.46) -> (69.31, 28.095)
  arc A381 (69.3369, 28.1219) -> (69.2831, 28.0681) centre (69.31, 28.095) ccw
  arc A382 (69.9181, 27.4331) -> (69.9719, 27.4869) centre (69.945, 27.46) ccw
  line L158 (69.31, 29.365) -> (69.945, 30)
  arc A383 (69.9719, 29.9731) -> (69.9181, 30.0269) centre (69.945, 30) ccw
  arc A384 (69.2831, 29.3919) -> (69.3369, 29.3381) centre (69.31, 29.365) ccw
  line L159 (71.215, 30) -> (69.945, 30)
  arc A385 (69.945, 30.0381) -> (69.945, 29.9619) centre (69.945, 30) ccw
  arc A386 (71.215, 29.9619) -> (71.215, 30.0381) centre (71.215, 30) ccw
  line L160 (74.39, 28.095) -> (75.025, 27.46)
  arc A387 (74.9981, 27.4331) -> (75.0519, 27.4869) centre (75.025, 27.46) ccw
  arc A388 (74.4169, 28.1219) -> (74.3631, 28.0681) centre (74.39, 28.095) ccw
  line L161 (75.025, 27.46) -> (76.295, 27.46)
  arc A389 (76.295, 27.4219) -> (76.295, 27.4981) centre (76.295, 27.46) ccw
  arc A390 (75.025, 27.4981) -> (75.025, 27.4219) centre (75.025, 27.46) ccw
  line L162 (76.295, 27.46) -> (76.93, 28.095)
  arc A391 (76.9569, 28.0681) -> (76.9031, 28.1219) centre (76.93, 28.095) ccw
  arc A392 (76.2681, 27.4869) -> (76.3219, 27.4331) centre (76.295, 27.46) ccw
  line L163 (76.93, 29.365) -> (76.295, 30)
  arc A393 (76.3219, 30.0269) -> (76.2681, 29.9731) centre (76.295, 30) ccw
  arc A394 (76.9031, 29.3381) -> (76.9569, 29.3919) centre (76.93, 29.365) ccw
  line L164 (76.295, 30) -> (75.025, 30)
  arc A395 (75.025, 30.0381) -> (75.025, 29.9619) centre (75.025, 30) ccw
  arc A396 (76.295, 29.9619) -> (76.295, 30.0381) centre (76.295, 30) ccw
  line L165 (75.025, 30) -> (74.39, 29.365)
  arc A397 (74.3631, 29.3919) -> (74.4169, 29.3381) centre (74.39, 29.365) ccw
  arc A398 (75.0519, 29.9731) -> (74.9981, 30.0269) centre (75.025, 30) ccw
  line L166 (76.93, 28.095) -> (77.565, 27.46)
  arc A399 (77.5381, 27.4331) -> (77.5919, 27.4869) centre (77.565, 27.46) ccw
  arc A400 (76.9569, 28.1219) -> (76.9031, 28.0681) centre (76.93, 28.095) ccw
  line L167 (77.565, 27.46) -> (78.835, 27.46)
  arc A401 (78.835, 27.4219) -> (78.835, 27.4981) centre (78.835, 27.46) ccw
  arc A402 (77.565, 27.4981) -> (77.565, 27.4219) centre (77.565, 27.46) ccw
  line L168 (79.47, 28.095) -> (79.47, 29.365)
  arc A403 (79.5081, 29.365) -> (79.4319, 29.365) centre (79.47, 29.365) ccw
  arc A404 (79.4319, 28.095) -> (79.5081, 28.095) centre (79.47, 28.095) ccw
  line L169 (78.835, 27.46) -> (79.47, 28.095)
  arc A405 (79.4969, 28.0681) -> (79.4431, 28.1219) centre (79.47, 28.095) ccw
  arc A406 (78.8081, 27.4869) -> (78.8619, 27.4331) centre (78.835, 27.46) ccw
  line L170 (79.47, 29.365) -> (78.835, 30)
  arc A407 (78.8619, 30.0269) -> (78.8081, 29.9731) centre (78.835, 30) ccw
  arc A408 (79.4431, 29.3381) -> (79.4969, 29.3919) centre (79.47, 29.365) ccw
  line L171 (78.835, 30) -> (77.565, 30)
  arc A409 (77.565, 30.0381) -> (77.565, 29.9619) centre (77.565, 30) ccw
  arc A410 (78.835, 29.9619) -> (78.835, 30.0381) centre (78.835, 30) ccw
  line L172 (77.565, 30) -> (76.93, 29.365)
  arc A411 (76.9031, 29.3919) -> (76.9569, 29.3381) centre (76.93, 29.365) ccw
  arc A412 (77.5919, 29.9731) -> (77.5381, 30.0269) centre (77.565, 30) ccw
  line L173 (47.9105, 31.3335) -> (47.593, 31.5875)
  arc A413 (47.6128, 31.6123) -> (47.5732, 31.5627) centre (47.593, 31.5875) ccw
  arc A414 (47.8907, 31.3087) -> (47.9303, 31.3583) centre (47.9105, 31.3335) ccw
  line L174 (47.593, 31.5875) -> (47.593, 30.4445)
  arc A415 (47.5613, 30.4445) -> (47.6248, 30.4445) centre (47.5931, 30.4445) ccw
  arc A416 (47.6248, 31.5875) -> (47.5613, 31.5875) centre (47.5931, 31.5875) ccw
  line L175 (47.9105, 30.4445) -> (47.2755, 30.4445)
  arc A417 (47.2755, 30.4763) -> (47.2755, 30.4128) centre (47.2755, 30.4445) ccw
  arc A418 (47.9105, 30.4128) -> (47.9105, 30.4763) centre (47.9105, 30.4445) ccw
  line L176 (78.8985, 26.7615) -> (78.581, 27.0155)
  arc A419 (78.6008, 27.0403) -> (78.5612, 26.9907) centre (78.581, 27.0155) ccw
  arc A420 (78.8787, 26.7367) -> (78.9183, 26.7863) centre (78.8985, 26.7615) ccw
  line L177 (78.581, 27.0155) -> (78.581, 25.8725)
  arc A421 (78.5493, 25.8725) -> (78.6128, 25.8725) centre (78.5811, 25.8725) ccw
  arc A422 (78.6128, 27.0155) -> (78.5493, 27.0155) centre (78.5811, 27.0155) ccw
  line L178 (78.8985, 25.8725) -> (78.2635, 25.8725)
  arc A423 (78.2635, 25.9043) -> (78.2635, 25.8408) centre (78.2635, 25.8726) ccw
  arc A424 (78.8985, 25.8408) -> (78.8985, 25.9043) centre (78.8985, 25.8726) ccw
  line L179 (77.7555, 25.8725) -> (77.438, 25.8725)
  arc A425 (77.438, 25.9043) -> (77.438, 25.8408) centre (77.438, 25.8726) ccw
  arc A426 (77.7555, 25.8408) -> (77.7555, 25.9043) centre (77.7555, 25.8726) ccw
  arc A427 (77.438, 26.5075) -> (77.438, 25.8725) centre (77.438, 26.19) ccw
  arc A428 (77.438, 26.4758) -> (77.438, 26.5392) centre (77.438, 26.5075) ccw
  arc A429 (77.438, 25.8408) -> (77.438, 25.9043) centre (77.438, 25.8726) ccw
  line L180 (77.7555, 27.0155) -> (77.3745, 27.0155)
  arc A430 (77.3745, 27.0473) -> (77.3745, 26.9838) centre (77.3745, 27.0155) ccw
  arc A431 (77.7555, 26.9838) -> (77.7555, 27.0473) centre (77.7555, 27.0155) ccw
  arc A432 (77.3745, 27.0155) -> (77.3745, 26.5075) centre (77.3745, 26.7615) ccw
  arc A433 (77.3745, 26.9838) -> (77.3745, 27.0473) centre (77.3745, 27.0155) ccw
  arc A434 (77.3745, 26.4758) -> (77.3745, 26.5392) centre (77.3745, 26.5075) ccw
  line L181 (77.3745, 26.5075) -> (77.6285, 26.5075)
  arc A435 (77.6285, 26.4758) -> (77.6285, 26.5392) centre (77.6285, 26.5075) ccw
  arc A436 (77.3745, 26.5392) -> (77.3745, 26.4758) centre (77.3745, 26.5075) ccw
  line L182 (92.13, 32.69) -> (92.13, 27.61)
  arc A437 (92.0983, 27.61) -> (92.1618, 27.61) centre (92.1301, 27.61) ccw
  arc A438 (92.1618, 32.69) -> (92.0983, 32.69) centre (92.1301, 32.69) ccw
  line L183 (92.13, 27.61) -> (90.86, 27.61)
  arc A439 (90.86, 27.6418) -> (90.86, 27.5783) centre (90.86, 27.6101) ccw
  arc A440 (92.13, 27.5783) -> (92.13, 27.6418) centre (92.13, 27.6101) ccw
  line L184 (90.86, 27.61) -> (83.24, 27.61)
  arc A441 (83.24, 27.6418) -> (83.24, 27.5783) centre (83.24, 27.6101) ccw
  arc A442 (90.86, 27.5783) -> (90.86, 27.6418) centre (90.86, 27.6101) ccw
  line L185 (83.24, 27.61) -> (81.97, 27.61)
  arc A443 (81.97, 27.6418) -> (81.97, 27.5783) centre (81.97, 27.6101) ccw
  arc A444 (83.24, 27.5783) -> (83.24, 27.6418) centre (83.24, 27.6101) ccw
  line L186 (81.97, 27.61) -> (81.97, 32.69)
  arc A445 (82.0018, 32.69) -> (81.9382, 32.69) centre (81.97, 32.69) ccw
  arc A446 (81.9382, 27.61) -> (82.0018, 27.61) centre (81.97, 27.61) ccw
  line L187 (81.97, 32.69) -> (92.13, 32.69)
  arc A447 (92.13, 32.6583) -> (92.13, 32.7218) centre (92.13, 32.69) ccw
  arc A448 (81.97, 32.7218) -> (81.97, 32.6583) centre (81.97, 32.69) ccw
  line L188 (90.86, 27.61) -> (90.86, 28.88)
  arc A449 (90.8918, 28.88) -> (90.8282, 28.88) centre (90.86, 28.88) ccw
  arc A450 (90.8282, 27.61) -> (90.8918, 27.61) centre (90.86, 27.61) ccw
  line L189 (90.86, 28.88) -> (83.24, 28.88)
  arc A451 (83.24, 28.9118) -> (83.24, 28.8483) centre (83.24, 28.88) ccw
  arc A452 (90.86, 28.8483) -> (90.86, 28.9118) centre (90.86, 28.88) ccw
  line L190 (83.24, 28.88) -> (83.24, 27.61)
  arc A453 (83.2083, 27.61) -> (83.2718, 27.61) centre (83.24, 27.61) ccw
  arc A454 (83.2718, 28.88) -> (83.2083, 28.88) centre (83.24, 28.88) ccw
  line L191 (35.695, 31.885) -> (36.695, 31.885)
  line L192 (36.695, 31.885) -> (36.695, 32.885)
  line L193 (36.695, 32.885) -> (35.695, 32.885)
  line L194 (35.695, 32.885) -> (35.695, 31.885)
  line L195 (33.6804, 33.3756) -> (33.6804, 31.3944)
  arc A455 (33.1851, 31.3944) -> (34.1757, 31.3944) centre (33.6804, 31.3944) ccw
  arc A456 (34.1757, 33.3756) -> (33.1851, 33.3756) centre (33.6804, 33.3756) ccw
  line L196 (33.6804, 33.3756) -> (33.6804, 31.3944)
  arc A457 (33.1851, 31.3944) -> (34.1757, 31.3944) centre (33.6804, 31.3944) ccw
  arc A458 (34.1757, 33.3756) -> (33.1851, 33.3756) centre (33.6804, 33.3756) ccw
  line L197 (38.7096, 33.3756) -> (38.7096, 31.3944)
  arc A459 (38.2143, 31.3944) -> (39.2049, 31.3944) centre (38.7096, 31.3944) ccw
  arc A460 (39.2049, 33.3756) -> (38.2143, 33.3756) centre (38.7096, 33.3756) ccw
  line L198 (38.7096, 33.3756) -> (38.7096, 31.3944)
  arc A461 (38.2143, 31.3944) -> (39.2049, 31.3944) centre (38.7096, 31.3944) ccw
  arc A462 (39.2049, 33.3756) -> (38.2143, 33.3756) centre (38.7096, 33.3756) ccw
  line L199 (50.006, 28.476) -> (50.514, 28.476)
  line L200 (50.514, 28.476) -> (50.514, 28.984)
  line L201 (50.514, 28.984) -> (50.006, 28.984)
  line L202 (50.006, 28.984) -> (50.006, 28.476)
  line L203 (47.466, 28.476) -> (47.974, 28.476)
  line L204 (47.974, 28.476) -> (47.974, 28.984)
  line L205 (47.974, 28.984) -> (47.466, 28.984)
  line L206 (47.466, 28.984) -> (47.466, 28.476)
  line L207 (52.546, 28.476) -> (53.054, 28.476)
  line L208 (53.054, 28.476) -> (53.054, 28.984)
  line L209 (53.054, 28.984) -> (52.546, 28.984)
  line L210 (52.546, 28.984) -> (52.546, 28.476)
  line L211 (57.626, 28.476) -> (58.134, 28.476)
  line L212 (58.134, 28.476) -> (58.134, 28.984)
  line L213 (58.134, 28.984) -> (57.626, 28.984)
  line L214 (57.626, 28.984) -> (57.626, 28.476)
  line L215 (55.086, 28.476) -> (55.594, 28.476)
  line L216 (55.594, 28.476) -> (55.594, 28.984)
  line L217 (55.594, 28.984) -> (55.086, 28.984)
  line L218 (55.086, 28.984) -> (55.086, 28.476)
  line L219 (60.166, 28.476) -> (60.674, 28.476)
  line L220 (60.674, 28.476) -> (60.674, 28.984)
  line L221 (60.674, 28.984) -> (60.166, 28.984)
  line L222 (60.166, 28.984) -> (60.166, 28.476)
  line L223 (65.246, 28.476) -> (65.754, 28.476)
  line L224 (65.754, 28.476) -> (65.754, 28.984)
  line L225 (65.754, 28.984) -> (65.246, 28.984)
  line L226 (65.246, 28.984) -> (65.246, 28.476)
  line L227 (62.706, 28.476) -> (63.214, 28.476)
  line L228 (63.214, 28.476) -> (63.214, 28.984)
  line L229 (63.214, 28.984) -> (62.706, 28.984)
  line L230 (62.706, 28.984) -> (62.706, 28.476)
  line L231 (67.786, 28.476) -> (68.294, 28.476)
  line L232 (68.294, 28.476) -> (68.294, 28.984)
  line L233 (68.294, 28.984) -> (67.786, 28.984)
  line L234 (67.786, 28.984) -> (67.786, 28.476)
  line L235 (72.866, 28.476) -> (73.374, 28.476)
  line L236 (73.374, 28.476) -> (73.374, 28.984)
  line L237 (73.374, 28.984) -> (72.866, 28.984)
  line L238 (72.866, 28.984) -> (72.866, 28.476)
  line L239 (70.326, 28.476) -> (70.834, 28.476)
  line L240 (70.834, 28.476) -> (70.834, 28.984)
  line L241 (70.834, 28.984) -> (70.326, 28.984)
  line L242 (70.326, 28.984) -> (70.326, 28.476)
  line L243 (75.406, 28.476) -> (75.914, 28.476)
  line L244 (75.914, 28.476) -> (75.914, 28.984)
  line L245 (75.914, 28.984) -> (75.406, 28.984)
  line L246 (75.406, 28.984) -> (75.406, 28.476)
  line L247 (77.946, 28.476) -> (78.454, 28.476)
  line L248 (78.454, 28.476) -> (78.454, 28.984)
  line L249 (78.454, 28.984) -> (77.946, 28.984)
  line L250 (77.946, 28.984) -> (77.946, 28.476)
  arc A463 (47.339, 28.73) -> (48.101, 28.73) centre (47.72, 28.73) ccw
  arc A464 (48.101, 28.73) -> (47.339, 28.73) centre (47.72, 28.73) ccw
  arc A465 (47.339, 28.73) -> (48.101, 28.73) centre (47.72, 28.73) ccw
  arc A466 (48.101, 28.73) -> (47.339, 28.73) centre (47.72, 28.73) ccw
  arc A467 (49.879, 28.73) -> (50.641, 28.73) centre (50.26, 28.73) ccw
  arc A468 (50.641, 28.73) -> (49.879, 28.73) centre (50.26, 28.73) ccw
  arc A469 (49.879, 28.73) -> (50.641, 28.73) centre (50.26, 28.73) ccw
  arc A470 (50.641, 28.73) -> (49.879, 28.73) centre (50.26, 28.73) ccw
  arc A471 (52.419, 28.73) -> (53.181, 28.73) centre (52.8, 28.73) ccw
  arc A472 (53.181, 28.73) -> (52.419, 28.73) centre (52.8, 28.73) ccw
  arc A473 (52.419, 28.73) -> (53.181, 28.73) centre (52.8, 28.73) ccw
  arc A474 (53.181, 28.73) -> (52.419, 28.73) centre (52.8, 28.73) ccw
  arc A475 (54.959, 28.73) -> (55.721, 28.73) centre (55.34, 28.73) ccw
  arc A476 (55.721, 28.73) -> (54.959, 28.73) centre (55.34, 28.73) ccw
  arc A477 (54.959, 28.73) -> (55.721, 28.73) centre (55.34, 28.73) ccw
  arc A478 (55.721, 28.73) -> (54.959, 28.73) centre (55.34, 28.73) ccw
  arc A479 (57.499, 28.73) -> (58.261, 28.73) centre (57.88, 28.73) ccw
  arc A480 (58.261, 28.73) -> (57.499, 28.73) centre (57.88, 28.73) ccw
  arc A481 (57.499, 28.73) -> (58.261, 28.73) centre (57.88, 28.73) ccw
  arc A482 (58.261, 28.73) -> (57.499, 28.73) centre (57.88, 28.73) ccw
  arc A483 (60.039, 28.73) -> (60.801, 28.73) centre (60.42, 28.73) ccw
  arc A484 (60.801, 28.73) -> (60.039, 28.73) centre (60.42, 28.73) ccw
  arc A485 (60.039, 28.73) -> (60.801, 28.73) centre (60.42, 28.73) ccw
  arc A486 (60.801, 28.73) -> (60.039, 28.73) centre (60.42, 28.73) ccw
  arc A487 (62.579, 28.73) -> (63.341, 28.73) centre (62.96, 28.73) ccw
  arc A488 (63.341, 28.73) -> (62.579, 28.73) centre (62.96, 28.73) ccw
  arc A489 (62.579, 28.73) -> (63.341, 28.73) centre (62.96, 28.73) ccw